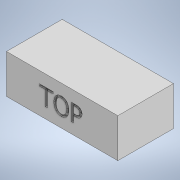
# Autodesk Inventor part: cable_jig_sevenmm_shim
Saved by Autodesk Inventor 2022 (Build 260153000, 153)
## iProperties
Created: 2022-03-09
Part Number: cable_jig_sevenmm_shim
Material: Generic
Document SubType Name: Modeling
Designer: kylem
Density: 1 g/cm^3
Appearance: Default
Author: kylem
Autodesk Inventor part; units mm, degrees
ref_plane "YZ Plane" through (0, 0, 0) normal (1, 0, 0) x (0, 1, 0)
ref_plane "XZ Plane" through (0, 0, 0) normal (0, 1, 0) x (-1, 0, 0)
ref_plane "XY Plane" through (0, 0, 0) normal (0, 0, 1) x (1, 0, 0)
sketch "Sketch1" plane through (0, 0, 0) normal (0, 1, 0) x (-1, 0, 0)
  line L0 (0, 0) -> (20, 0)
  line L1 (20, 0) -> (20, -10)
  line L2 (20, -10) -> (0, -10)
  line L3 (0, -10) -> (0, 0)
  dimension "d0" = 20
  dimension "d1" = 10
  constraints: 8 end point, 2 parallel, 1 horizontal, 1 perpendicular
  measures "d0" distance of L1.end L2.end
  measures "d1" distance of L0.end L1.end
extrude "Extrusion1" add sketch "Sketch1" along normal blind 7
sketch "Sketch2" plane through (-20, 0, 0) normal (0, 0, 1) x (1, 0, 0)
  line L0 (5.9298, 5.0041) -> (16.3941, 5.0041) construction
  line L1 (16.3941, 5.0041) -> (16.3941, 1.9722) construction
  line L2 (16.3941, 1.9722) -> (5.9298, 1.9722) construction
  line L3 (5.9298, 1.9722) -> (5.9298, 5.0041) construction
  line L4 (6.9499, 1.8918) -> (6.9499, 4.5792)
  line L5 (6.9499, 4.5792) -> (5.9273, 4.5792)
  line L6 (5.9273, 4.5792) -> (5.9273, 4.9398)
  line L7 (5.9273, 4.9398) -> (8.3776, 4.9398)
  line L8 (8.3776, 4.9398) -> (8.3776, 4.5792)
  line L9 (8.3776, 4.5792) -> (7.355, 4.5792)
  line L10 (7.355, 4.5792) -> (7.355, 1.8918)
  line L11 (7.355, 1.8918) -> (6.9499, 1.8918)
  spline S0 degree 2 poles (10.8426, 4.5916) (11.0155, 4.389) (11.2082, 3.7962) (11.2082, 3.4158) knots 0 0 0 1 2 2 2
  spline S1 degree 2 poles (11.2082, 3.4158) (11.2082, 3.0453) (11.0205, 2.4451) (10.8426, 2.2426) knots 0 0 0 1 2 2 2
  spline S2 degree 2 poles (10.8426, 2.2426) (10.6549, 2.0302) (10.1584, 1.8276) (9.8596, 1.8276) knots 0 0 0 1 2 2 2
  spline S3 degree 2 poles (9.8596, 1.8276) (9.5508, 1.8276) (9.0568, 2.0376) (8.8765, 2.2426) knots 0 0 0 1 2 2 2
  spline S4 degree 2 poles (8.8765, 2.2426) (8.7011, 2.4451) (8.5134, 3.0404) (8.5134, 3.4158) knots 0 0 0 1 2 2 2
  spline S5 degree 2 poles (8.5134, 3.4158) (8.5134, 3.7987) (8.7036, 4.3816) (8.879, 4.5916) knots 0 0 0 1 2 2 2
  spline S6 degree 2 poles (8.879, 4.5916) (9.0568, 4.7941) (9.5533, 5.0041) (9.8596, 5.0041) knots 0 0 0 1 2 2 2
  spline S7 degree 2 poles (9.8596, 5.0041) (10.1708, 5.0041) (10.6697, 4.7867) (10.8426, 4.5916) knots 0 0 0 1 2 2 2
  spline S8 degree 2 poles (10.7858, 3.4158) (10.7858, 3.7172) (10.6549, 4.184) (10.5364, 4.3371) knots 0 0 0 1 2 2 2
  spline S9 degree 2 poles (10.5364, 4.3371) (10.4153, 4.4952) (10.0745, 4.6533) (9.862, 4.6533) knots 0 0 0 1 2 2 2
  spline S10 degree 2 poles (9.862, 4.6533) (9.6422, 4.6533) (9.3112, 4.5002) (9.1853, 4.3371) knots 0 0 0 1 2 2 2
  spline S11 degree 2 poles (9.1853, 4.3371) (9.0642, 4.1815) (8.9358, 3.7122) (8.9358, 3.4158) knots 0 0 0 1 2 2 2
  spline S12 degree 2 poles (8.9358, 3.4158) (8.9358, 2.8156) (9.4397, 2.1784) (9.862, 2.1784) knots 0 0 0 1 2 2 2
  spline S13 degree 2 poles (9.862, 2.1784) (10.2844, 2.1784) (10.7858, 2.8156) (10.7858, 3.4158) knots 0 0 0 1 2 2 2
  spline S14 degree 2 poles (13.5794, 4.021) (13.5794, 3.8234) (13.4386, 3.4677) (13.3127, 3.3442) knots 0 0 0 1 2 2 2
  spline S15 degree 2 poles (13.3127, 3.3442) (13.1546, 3.1886) (12.7273, 3.028) (12.4012, 3.028) knots 0 0 0 1 2 2 2
  line L12 (12.4012, 3.028) -> (12.0579, 3.028)
  line L13 (12.0579, 3.028) -> (12.0579, 1.8918)
  line L14 (12.0579, 1.8918) -> (11.6528, 1.8918)
  line L15 (11.6528, 1.8918) -> (11.6528, 4.9398)
  line L16 (11.6528, 4.9398) -> (12.4185, 4.9398)
  spline S16 degree 2 poles (12.4185, 4.9398) (12.6902, 4.9398) (13.0706, 4.8509) (13.2163, 4.7496) knots 0 0 0 1 2 2 2
  spline S17 degree 2 poles (13.2163, 4.7496) (13.3868, 4.6336) (13.5794, 4.2754) (13.5794, 4.021) knots 0 0 0 1 2 2 2
  spline S18 degree 2 poles (13.157, 4.0086) (13.157, 4.1667) (13.0484, 4.3989) (12.9372, 4.473) knots 0 0 0 1 2 2 2
  spline S19 degree 2 poles (12.9372, 4.473) (12.8409, 4.5372) (12.584, 4.5891) (12.3938, 4.5891) knots 0 0 0 1 2 2 2
  line L17 (12.3938, 4.5891) -> (12.0579, 4.5891)
  line L18 (12.0579, 4.5891) -> (12.0579, 3.3738)
  line L19 (12.0579, 3.3738) -> (12.3345, 3.3738)
  spline S20 degree 2 poles (12.3345, 3.3738) (12.5815, 3.3738) (12.8853, 3.4529) (12.9841, 3.5566) knots 0 0 0 1 2 2 2
  spline S21 degree 2 poles (12.9841, 3.5566) (13.0755, 3.648) (13.157, 3.8629) (13.157, 4.0086) knots 0 0 0 1 2 2 2
  point P0 (20, 0)
  constraints: 2 other
extrude "Extrusion3" cut sketch "Sketch2" against normal blind 0.5
body "Solid1"
